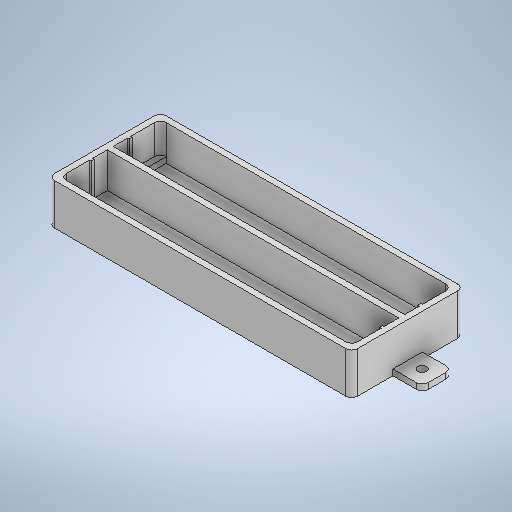
# Autodesk Inventor part: power_strip
Saved by Autodesk Inventor 2025.1 (Build 291241000, 241)
## iProperties
Created: 2025-04-10
Part Number: power_strip
Material: Generic
Document SubType Name: Modeling
Designer: Ian Ching
Density: 1 g/cm^3
Appearance: Default
Author: Ian Ching
Autodesk Inventor part; units mm, degrees
ref_plane "YZ Plane" through (0, 0, 0) normal (1, 0, 0) x (0, 1, 0)
ref_plane "XZ Plane" through (0, 0, 0) normal (0, 1, 0) x (-1, 0, 0)
ref_plane "XY Plane" through (0, 0, 0) normal (0, 0, 1) x (1, 0, 0)
sketch "Sketch1" plane through (0, 0, 0) normal (0, 1, 0) x (-1, 0, 0)
  line L0 (0, 0) -> (-103, 0)
  line L1 (-103, 0) -> (-103, -38)
  line L2 (-103, -38) -> (0, -38)
  line L3 (0, -38) -> (0, 0)
  dimension "d0" = 103
  dimension "d1" = 38
  constraints: 8 end point, 2 parallel, 1 horizontal, 1 perpendicular
  measures "d0" distance of L2.end L1.end
  measures "d1" distance of L1.end L0.end
extrude "Extrusion1" add sketch "Sketch1" along normal blind 2
sketch "Sketch2" plane through (0, 2, 0) normal (0, 1, 0) x (1, 0, 0)
  line L0 (2, 2) -> (101, 2)
  line L1 (101, 2) -> (101, 18)
  line L2 (101, 18) -> (2, 18)
  line L3 (2, 18) -> (2, 2)
  line L4 (2, 20) -> (101, 20)
  line L5 (101, 20) -> (101, 36)
  line L6 (101, 36) -> (2, 36)
  line L7 (2, 36) -> (2, 20)
  line L8 (0, 0) -> (2, 0)
  line L9 (2, 0) -> (2, 2)
  line L10 (2, 2) -> (0, 2)
  line L11 (0, 2) -> (0, 0)
  line L12 (103, 38) -> (0, 38) projected
  line L13 (0, 38) -> (2, 38)
  line L14 (2, 38) -> (2, 36)
  line L15 (2, 36) -> (0, 36)
  line L16 (0, 36) -> (0, 38)
  line L17 (103, 0) -> (103, 38) projected
  line L18 (0, 0) -> (103, 0)
  line L19 (103, 0) -> (103, 38)
  line L20 (103, 38) -> (0, 38)
  line L21 (0, 38) -> (0, 0)
  dimension "d4" = 99
  dimension "d5" = 16
  dimension "d6" = 99
  dimension "d7" = 16
  dimension "d8" = 2
  dimension "d9" = 2
  dimension "d10" = 2
  dimension "d11" = 2
  constraints: 40 end point, 10 parallel, 5 horizontal, 5 perpendicular
  measures "d4" distance of L2.end L1.end
  measures "d5" distance of L1.end L0.end
  measures "d6" distance of L6.end L5.end
  measures "d7" distance of L5.end L4.end
  measures "d8" distance of L10.end L0.start
  measures "d9" distance of L0.start L8.end
  measures "d10" distance of L6.end L15.end
  measures "d11" distance of L13.end L6.end
extrude "Extrusion2" add sketch "Sketch2" along normal blind 12
sketch "Sketch3" plane through (101, 2, -18) normal (-1, 0, 0) x (0, 0, 1)
  line L0 (18, 12) -> (-20, 12) projected
  line L1 (5, 12) -> (6, 12)
  line L2 (6, 12) -> (6, 0)
  line L3 (6, 0) -> (5, 0)
  line L4 (5, 0) -> (5, 12)
  line L5 (0, 12) -> (5, 12)
  line L6 (5, 12) -> (5, 0)
  line L7 (5, 0) -> (0, 0)
  line L8 (0, 0) -> (0, 12)
  point P0 (18, -2)
  dimension "d14" = 1
  dimension "d15" = 12
  dimension "d16" = 5
  dimension "d17" = 12
  constraints: 16 end point, 4 parallel, 2 horizontal, 2 perpendicular, 2 point on line
  measures "d14" distance of L2.end L3.end
  measures "d15" distance of L1.end L2.end
  measures "d16" distance of L6.end L7.end
  measures "d17" distance of L1.start L6.end
extrude "Extrusion3" add sketch "Sketch3" along normal blind 0.5 contours L2 L3 L4 L0
sketch "Sketch4" plane through (2, 2, -2) normal (1, 0, 0) x (0, 0, -1)
  line L0 (16, 12) -> (11, 12)
  line L1 (11, 12) -> (11, 0)
  line L2 (11, 0) -> (16, 0)
  line L3 (16, 0) -> (16, 12)
  line L4 (11, 12) -> (10, 12)
  line L5 (10, 12) -> (10, 0)
  line L6 (10, 0) -> (11, 0)
  line L7 (11, 0) -> (11, 12)
  point P0 (-2, -2)
  point P1 (11, 0)
  dimension "d20" = 5
  dimension "d21" = 12
  dimension "d22" = 1
  dimension "d23" = 12
  constraints: 16 end point, 4 parallel, 2 horizontal, 2 perpendicular
  measures "d20" distance of L2.end L1.end
  measures "d21" distance of L1.end L0.end
  measures "d22" distance of L6.end L5.end
  measures "d23" distance of L5.end L4.end
extrude "Extrusion4" add sketch "Sketch4" along normal blind 0.5 contours L1 L6 L5 L4
sketch "Sketch5" plane through (2, 2, -20) normal (1, 0, 0) x (0, 0, -1)
  line L0 (0, 12) -> (5, 12)
  line L1 (5, 12) -> (5, 0)
  line L2 (5, 0) -> (0, 0)
  line L3 (0, 0) -> (0, 12)
  line L4 (5, 12) -> (6, 12)
  line L5 (6, 12) -> (6, 0)
  line L6 (6, 0) -> (5, 0)
  line L7 (5, 0) -> (5, 12)
  point P0 (-20, -2)
  point P1 (5, 0)
  dimension "d26" = 5
  dimension "d27" = 12
  dimension "d28" = 1
  dimension "d29" = 12
  constraints: 16 end point, 4 parallel, 2 horizontal, 2 perpendicular
  measures "d26" distance of L1.end L2.end
  measures "d27" distance of L0.end L1.end
  measures "d28" distance of L5.end L6.end
  measures "d29" distance of L4.end L5.end
extrude "Extrusion5" add sketch "Sketch5" along normal blind 0.5 contours L4 L5 L6 L1
sketch "Sketch6" plane through (101, 2, -36) normal (-1, 0, 0) x (0, 0, 1)
  line L0 (16, 12) -> (11, 12)
  line L1 (11, 12) -> (11, 0)
  line L2 (11, 0) -> (16, 0)
  line L3 (16, 0) -> (16, 12)
  line L4 (11, 12) -> (10, 12)
  line L5 (10, 12) -> (10, 0)
  line L6 (10, 0) -> (11, 0)
  line L7 (11, 0) -> (11, 12)
  point P0 (36, -2)
  point P1 (11, 0)
  dimension "d32" = 5
  dimension "d33" = 12
  dimension "d34" = 1
  dimension "d35" = 12
  constraints: 16 end point, 4 parallel, 2 horizontal, 2 perpendicular
  measures "d32" distance of L2.end L1.end
  measures "d33" distance of L1.end L0.end
  measures "d34" distance of L6.end L5.end
  measures "d35" distance of L5.end L4.end
extrude "Extrusion6" add sketch "Sketch6" along normal blind 0.5 contours L1 L6 L5 L4
sketch "Sketch7" plane through (103, 0, 0) normal (1, 0, 0) x (0, 0, -1)
  line L0 (14, 0) -> (24, 0)
  line L1 (24, 0) -> (24, 2)
  line L2 (24, 2) -> (14, 2)
  line L3 (14, 2) -> (14, 0)
  line L4 (0, 0) -> (38, 0) projected
  point P0 (19, 0)
  dimension "d38" = 10
  dimension "d39" = 2
  constraints: 8 end point, 2 midpoint, 2 parallel, 1 horizontal, 1 perpendicular
  measures "d38" distance of L2.end L1.end
  measures "d39" distance of L1.end L0.end
extrude "Extrusion7" add sketch "Sketch7" along normal blind 10
sketch "Sketch8" plane through (103, 2, -14) normal (0, 1, 0) x (1, 0, 0)
  line L0 (10, 10) -> (10, 0) projected
  line L1 (10, 5) -> (0, 5)
  line L2 (0, -14) -> (0, 24) projected
  circle A0 centre (5, 5) radius 1.5
  point P0 (-103, -14)
  dimension "d42" = 3
  constraints: 3 midpoint, 2 end point, 1 centre point
  measures "d42" diameter of A0
extrude "Extrusion8" cut sketch "Sketch8" against normal blind 2
sketch "Sketch9" plane through (0, 0, -38) normal (-1, 0, 0) x (0, 0, 1)
  line L0 (24, 0) -> (14, 0)
  line L1 (14, 0) -> (14, 2)
  line L2 (14, 2) -> (24, 2)
  line L3 (24, 2) -> (24, 0)
  line L4 (0, 0) -> (38, 0) projected
  point P0 (19, 0)
  dimension "d45" = 10
  dimension "d46" = 2
  constraints: 8 end point, 2 midpoint, 2 parallel, 1 horizontal, 1 perpendicular
  measures "d45" distance of L1.end L2.end
  measures "d46" distance of L0.end L1.end
extrude "Extrusion9" add sketch "Sketch9" along normal blind 10
sketch "Sketch10" plane through (0, 2, -14) normal (0, 1, 0) x (1, 0, 0)
  line L0 (-10, 10) -> (-10, 0) projected
  line L1 (-10, 5) -> (0, 5)
  line L2 (0, 24) -> (0, -14) projected
  circle A0 centre (-5, 5) radius 1.5
  dimension "d49" = 3
  constraints: 3 midpoint, 2 end point, 1 centre point
  measures "d49" diameter of A0
extrude "Extrusion10" cut sketch "Sketch10" against normal blind 2
fillet "Fillet1" radius 2 12 edges at (0, 7, 0) (103, 7, 0) (103, 7, -38) (113, 1, -14) (113, 1, -24) (0, 7, -38) (-10, 1, -24) (-10, 1, -14) (2, 8, -36) (101, 8, -36) (101, 8, -2) (2, 8, -2)
sketch "Sketch11" plane through (0, 2, 0) normal (0, 1, 0) x (1, 0, 0)
  line L0 (101, 36) -> (99, 36)
  line L1 (99, 36) -> (99, 29.4)
  line L2 (99, 29.4) -> (101, 29.4)
  line L3 (101, 29.4) -> (101, 36)
  line L4 (2, 36) -> (4, 36)
  line L5 (4, 36) -> (4, 29.4)
  line L6 (4, 29.4) -> (2, 29.4)
  line L7 (2, 29.4) -> (2, 36)
  line L8 (2, 2) -> (4, 2)
  line L9 (4, 2) -> (4, 8.6)
  line L10 (4, 8.6) -> (2, 8.6)
  line L11 (2, 8.6) -> (2, 2)
  line L12 (101, 2) -> (99, 2)
  line L13 (99, 2) -> (99, 8.6)
  line L14 (99, 8.6) -> (101, 8.6)
  line L15 (101, 8.6) -> (101, 2)
  point P0 (0, 0)
  dimension "d53" = 2
  dimension "d54" = 6.6
  dimension "d55" = 2
  dimension "d56" = 6.6
  dimension "d57" = 2
  dimension "d58" = 6.6
  dimension "d59" = 2
  dimension "d60" = 6.6
  constraints: 32 end point, 8 parallel, 4 horizontal, 4 perpendicular, 2 point on line
  measures "d53" distance of L2.end L1.end
  measures "d54" distance of L1.end L0.end
  measures "d55" distance of L5.end L6.end
  measures "d56" distance of L4.end L5.end
  measures "d57" distance of L10.end L9.end
  measures "d58" distance of L9.end L8.end
  measures "d59" distance of L13.end L14.end
  measures "d60" distance of L12.end L13.end
extrude "Extrusion11" add sketch "Sketch11" along normal blind 2
body "Solid1"
